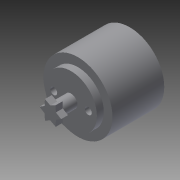
# Autodesk Inventor part: 000109
Saved by Autodesk Inventor 2015 (Build 190159000, 159)
## iProperties
Created: 2015-05-13
Part Number: 000109
Material: Generic
Document SubType Name: Modeling
Designer: Angelina
Density: 1 g/cm^3
Appearance: Default
Author: Angelina
Autodesk Inventor part; units mm, degrees
ref_plane "YZ Plane" through (0, 0, 0) normal (1, 0, 0) x (0, 1, 0)
ref_plane "XZ Plane" through (0, 0, 0) normal (0, 1, 0) x (-1, 0, 0)
sketch "Sketch1" plane through (0, 0, 0) normal (0, 0, 1) x (1, 0, 0)
  circle A0 centre (0, 0) radius 12.7
  dimension "d0" = 25.4
  constraints: 1 centre point, 1 coincident
  measures "d0" diameter of A0
extrude "Extrusion1" add sketch "Sketch1" along normal blind 19.05
sketch "Sketch2" plane through (0, 0, 19.05) normal (0, 0, 1) x (1, 0, 0)
  circle A0 centre (0, 0) radius 9.525
  dimension "d3" = 19.05
  constraints: 1 centre point, 1 coincident
  measures "d3" diameter of A0
extrude "Extrusion2" add sketch "Sketch2" along normal blind 1.27
sketch "Sketch3" plane through (0, 0, 20.32) normal (0, 0, 1) x (1, 0, 0)
  circle A0 centre (0, 0) radius 9.525
  dimension "d6" = 19.05
  constraints: 1 centre point, 1 coincident
  measures "d6" diameter of A0
extrude "Extrusion3" add sketch "Sketch3" along normal blind 1.27
sketch "Sketch4" plane through (0, 0, 21.59) normal (0, 0, 1) x (1, 0, 0)
  circle A0 centre (0, 0) radius 2.3729
  constraints: 1 centre point, 1 coincident
extrude "Extrusion4" add sketch "Sketch4" along normal blind 5.08
ref_plane "Work Plane1" through (0, 0, 26.67) normal (0, 0, 1) x (1, 0, 0)
sketch "Sketch10" plane through (0, 0, 26.67) normal (0, 0, 1) x (1, 0, 0)
  circle A0 centre (0, 0) radius 2.3813 construction
  circle A1 centre (0, 0) radius 3.9688 construction
  line L0 (0, 4.2939) -> (0, -5.5705) construction
  line L1 (6.3712, 0) -> (-7.3964, 0) construction
  line L2 (0, 2.3813) -> (1.9844, 3.437)
  line L3 (1.9844, 3.437) -> (2.0622, 1.1906)
  line L4 (-2.0622, 1.1906) -> (-1.9844, 3.437)
  line L5 (-1.9844, 3.437) -> (0, 2.3813)
  line L6 (-2.0622, -1.1906) -> (-3.9688, 0)
  line L7 (-3.9688, 0) -> (-2.0622, 1.1906)
  line L8 (0, -2.3813) -> (-1.9844, -3.437)
  line L9 (-1.9844, -3.437) -> (-2.0622, -1.1906)
  line L10 (2.0622, -1.1906) -> (1.9844, -3.437)
  line L11 (1.9844, -3.437) -> (0, -2.3813)
  line L12 (2.0622, 1.1906) -> (3.9688, 0)
  line L13 (3.9688, 0) -> (2.0622, -1.1906)
  line L14 (-2.0622, -1.1906) -> (0, -2.3813)
  line L15 (0, -2.3813) -> (2.0622, -1.1906)
  line L16 (2.0622, -1.1906) -> (2.0622, 1.1906)
  line L17 (2.0622, 1.1906) -> (0, 2.3813)
  line L18 (0, 2.3813) -> (-2.0622, 1.1906)
  line L19 (-2.0622, 1.1906) -> (-2.0622, -1.1906)
  line L20 (-2.0622, 1.1906) -> (0, 2.3813)
  line L21 (2.0622, 1.1906) -> (0, 2.3813)
  line L22 (2.0622, 1.1906) -> (2.0622, -1.1906)
  line L23 (2.0622, -1.1906) -> (0, -2.3813)
  line L24 (0, -2.3813) -> (-2.0622, -1.1906)
  line L25 (-2.0622, -1.1906) -> (-2.0622, 1.1906)
  line L26 (-3.9688, 0) -> (-2.0622, 1.1906)
  line L27 (-2.0622, -1.1906) -> (-2.0622, 1.1906)
  line L28 (-2.0622, -1.1906) -> (-3.9688, 0)
  line L29 (0, -2.3813) -> (-1.9844, -3.437)
  line L30 (-1.9844, -3.437) -> (-2.0622, -1.1906)
  line L31 (-2.0622, -1.1906) -> (0, -2.3812)
  line L32 (2.0622, -1.1906) -> (1.9844, -3.437)
  line L33 (1.9844, -3.437) -> (0, -2.3813)
  line L34 (0, -2.3812) -> (2.0622, -1.1906)
  line L35 (2.0622, 1.1906) -> (3.9688, 0)
  line L36 (3.9688, 0) -> (2.0622, -1.1906)
  line L37 (2.0622, -1.1906) -> (2.0622, 1.1906)
  line L38 (0, 2.3813) -> (1.9844, 3.437)
  line L39 (1.9844, 3.437) -> (2.0622, 1.1906)
  line L40 (2.0622, 1.1906) -> (0, 2.3813)
  line L41 (-2.0622, 1.1906) -> (-1.9844, 3.437)
  line L42 (-1.9844, 3.437) -> (0, 2.3813)
  line L43 (0, 2.3813) -> (-2.0622, 1.1906)
  line L44 (-2.0622, 1.1906) -> (0, 2.3813)
  line L45 (0, 2.3813) -> (-1.9844, 3.437)
  line L46 (-1.9844, 3.437) -> (-2.0622, 1.1906)
  line L47 (0, 2.3813) -> (1.9844, 3.437)
  line L48 (1.9844, 3.437) -> (2.0622, 1.1906)
  line L49 (0, 2.3813) -> (2.0622, 1.1906)
  line L50 (2.0622, 1.1906) -> (2.0622, -1.1906)
  line L51 (2.0622, -1.1906) -> (3.9688, 0)
  line L52 (3.9688, 0) -> (2.0622, 1.1906)
  line L53 (2.0622, -1.1906) -> (0, -2.3812)
  line L54 (0, -2.3812) -> (1.9844, -3.437)
  line L55 (1.9844, -3.437) -> (2.0622, -1.1906)
  line L56 (0, -2.3812) -> (-1.9844, -3.437)
  line L57 (-2.0622, -1.1906) -> (-1.9844, -3.437)
  line L58 (-2.0622, -1.1906) -> (0, -2.3812)
  line L59 (-2.0622, -1.1906) -> (-2.0622, 1.1906)
  line L60 (-2.0622, 1.1906) -> (-3.9688, 0)
  line L61 (-3.9688, 0) -> (-2.0622, -1.1906)
  point P0 (3.9688, 0)
  point P1 (-1.9844, 3.437)
  point P2 (-3.9688, 0)
  point P3 (-1.9844, -3.437)
  point P4 (1.9844, -3.437)
  dimension "d26" = 4.7625
  dimension "d27" = 7.9375
  dimension "d30" = 360
  dimension "d34" = 360
  dimension "d38" = 360
  dimension "d42" = 360
  constraints: 124 end point, 14 equal length, 4 point on line, 2 coincident, 1 horizontal, 1 horizontal alignment, 1 vertical, 1 vertical alignment, 116 other
extrude "Extrusion10" add sketch "Sketch10" along normal blind 2.54
sketch "Sketch11" plane through (0, 0, 21.59) normal (0, 0, 1) x (1, 0, 0)
  point P0 (0, 0)
  point P1 (-6.35, 0)
  point P2 (6.35, 0)
  dimension "d46" = 6.35
  dimension "d47" = 6.35
  measures "d46" distance of point (6.35, 0) point (0, 0)
  measures "d47" distance of point (0, 0) point (-6.35, 0)
hole "Hole1" at (-6.35, 0, 21.59) at (6.35, 0, 21.59) direction (0, 0, -1) diameter 2.54 depth 12.7 tip angle 118
body "Solid1"
